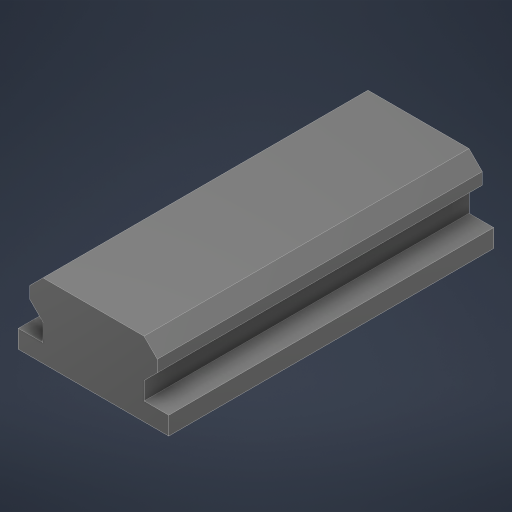
# Autodesk Inventor part: Picatinny model
Saved by Autodesk Inventor 2023 (Build 270158000, 158)
## iProperties
Created: 2023-10-16
Part Number: Picatinny model
Material: Generic
Document SubType Name: Modeling
Designer: nick_
Density: 1 g/cm^3
Appearance: Smooth - Black
Author: nick_
Autodesk Inventor part; units mm, degrees
ref_plane "YZ Plane" through (0, 0, 0) normal (1, 0, 0) x (0, 1, 0)
ref_plane "XZ Plane" through (0, 0, 0) normal (0, 1, 0) x (-1, 0, 0)
ref_plane "XY Plane" through (0, 0, 0) normal (0, 0, 1) x (1, 0, 0)
sketch "Sketch1" plane through (0, 0, 0) normal (0, 0, 1) x (1, 0, 0)
  line L0 (-12.5, 0) -> (-8.3947, 0)
  line L1 (-8.3947, 0) -> (-8.3947, 2.9464)
  line L2 (-8.3947, 2.9464) -> (-10.6045, 5.1562)
  line L3 (-10.6045, 5.1562) -> (-10.6045, 7.112)
  line L4 (-10.6045, 7.112) -> (-8.3947, 9.3218)
  line L5 (-8.3947, 9.3218) -> (0, 9.3218)
  line L6 (0, 9.3218) -> (0, -3)
  line L7 (0, -3) -> (-12.5, -3)
  line L8 (-12.5, -3) -> (-12.5, 0)
  point P0 (0, 0)
  point P1 (-9.4996, 4.0513)
  point P2 (-9.4996, 8.2169)
  dimension "d1" = 21.209
  dimension "d5" = 45
  dimension "d6" = 45
  dimension "d7" = 4.1656
  dimension "d9" = 18.9992
  dimension "d10" = 9.3218
  dimension "d11" = 25
  dimension "d12" = 3
  constraints: 18 end point, 5 perpendicular, 2 midpoint, 2 parallel, 1 horizontal, 1 horizontal alignment, 1 point on line
  measures "d1" diameter of L3 L6
  measures "d5" angle of L4 L3
  measures "d6" angle of L2 L3
  measures "d7" distance of point (-9.5, 4.051) point (-9.5, 8.217)
  measures "d9" diameter of point (-9.5, 8.217) L6
  measures "d10" distance between parallel lines of L0 L5
  measures "d11" diameter of L8 L6
  measures "d12" distance of L7.end L0.start
extrude "Extrusion1" add sketch "Sketch1" along normal blind 54
mirror "Mirror1" about plane through (0, -3, 0) normal (1, 0, 0) of "Extrusion1"
body "Solid1"
